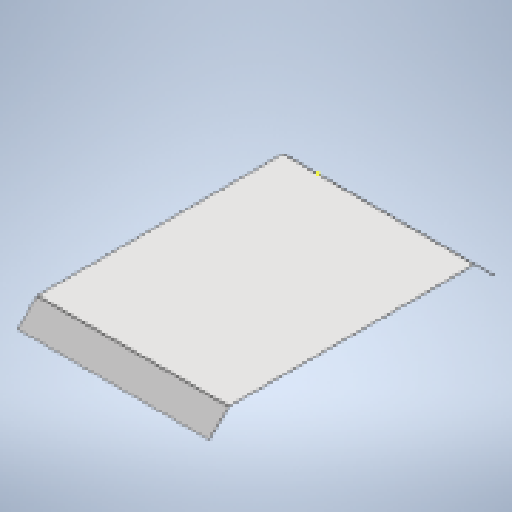
# Autodesk Inventor part: BSH 010 floor 1
Saved by Autodesk Inventor 2025 (Build 290162010, 162A)
## iProperties
Created: 2024-07-23
Part Number: BSH 010 floor 1
Material: 09g2s
Document SubType Name: Sheet Metal
Designer: admin
Density: 7.85 g/cm^3
Sheet Metal Rule: AISI304 3mm Die 32
Appearance: Default
Flat Pattern Width: 148 cm
Flat Pattern Length: 232.067 cm
Flat Pattern Area: 34346 cm^2
Sheet Metal Width: 1480,000 mm
Sheet Metal Length: 2320,673 mm
Sheet Metal Area: 3434595,446 mm^2
Author: admin
Autodesk Inventor part; units mm, degrees
ref_plane "YZ Plane" through (0, 0, 0) normal (1, 0, 0) x (0, 1, 0)
ref_plane "XZ Plane" through (0, 0, 0) normal (0, 1, 0) x (-1, 0, 0)
ref_plane "XY Plane" through (0, 0, 0) normal (0, 0, 1) x (1, 0, 0)
sketch "Sketch1" plane through (0, 0, 0) normal (0, 0, 1) x (1, 0, 0)
  line L0 (-740, -950) -> (740, -950)
  line L1 (740, -950) -> (740, 950)
  line L2 (740, 950) -> (-740, 950)
  line L3 (-740, 950) -> (-740, -950)
  line L4 (-740, -950) -> (740, 950) construction
  line L5 (740, -950) -> (-740, 950) construction
  point P0 (0, 0)
  dimension "d0" = 1480
  dimension "d1" = 1900
  measures "d0" distance of L2.end L1.end
  measures "d1" distance of L1.end L0.end
extrude "Plate1" add sketch "Sketch1" along normal blind 3
sketch "Sketch2" plane through (740, 947.8787, 0.8787) normal (0, 0.7071068, 0.7071068) x (-1, 0, 0)
  line L0 (1480, 0) -> (0, 0)
  line L1 (0, 0) -> (0, -212)
  line L2 (0, -212) -> (1480, -212)
  line L3 (1480, -212) -> (1480, 0)
  constraints: 6 end point, 1 horizontal, 1 perpendicular, 1 vertical
edge flange "Flange1" height 212 angle 45 thickness 3 bend radius 5 thickness toward (0, 0.7071068, 0.7071068) relief round relief width 3 relief depth 1.5 corner gap 5 corner form 0 edges at (0, 950, 0) (0, -950, 0) wall of the first edge with corners at (-740, 947.8787, 0.8787) (740, 947.8787, 0.8787) (740, 1097.7853, -149.028) (-740, 1097.7853, -149.028)
bend "Bend1"
corner "Corner1"
sketch "Sketch3" plane through (740, 1097.7853, -149.028) normal (0, -0.7071068, -0.7071068) x (-1, 0, 0)
  point P0 (740, -881.6301)
sketch "Sketch4" plane through (740, 1097.7853, -149.028) normal (0, -0.7071068, -0.7071068) x (-1, 0, 0)
  line L0 (25, -40) -> (25, -25) construction
  line L1 (25, -25) -> (225, -25) construction
  line L2 (225, -25) -> (225, -40) construction
  line L3 (225, -40) -> (25, -40) construction
  line L4 (1480, 0) -> (0, 0) projected
  line L5 (0, -208.6863) -> (0, 0) projected
  point P0 (740, -881.6301)
  dimension "d13" = 200
  dimension "d14" = 15
  dimension "d15" = 25
  dimension "d16" = 25
  constraints: 2 other
  measures "d13" distance of L0.end L1.end
  measures "d14" distance between parallel lines of L1 L3
  measures "d15" distance between parallel lines of L4 L1
  measures "d16" distance between parallel lines of L5 L0
mark "Mark1"
equation "\"d2\" = Thickness"
equation "\"d3\" = BendReliefWidth"
equation "\"d4\" = BendReliefDepth"
equation "\"d5\" = MinimumRemnant"
equation "\"d6\" = TransitionRadius"
equation "\"d9\" = BendRadius"
equation "\"d10\" = CornerReliefSize"
equation "\"d11\" = GapSize"
equation "\"d12\" = JacobiRadiusSize"
equation "\"BendReliefWidth\" = Thickness"
equation "\"BendReliefDepth\" = 0.5 * Thickness"
equation "\"CornerReliefSize\" = 4 * Thickness"
equation "\"MinimumRemnant\" = 2 * Thickness"
equation "\"TransitionRadius\" = BendRadius"
equation "\"JacobiRadiusSize\" = BendRadius"
equation "\"GapSize\" = Thickness"
equation "\"Thickness\" = 3"
equation "\"BendRadius\" = 5"
body "Solid1"
